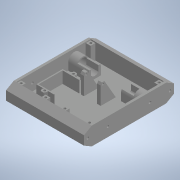
# Autodesk Inventor part: HexBody
Saved by Autodesk Inventor 2020 (Build 240168000, 168)
## iProperties
Created: 2023-12-19
Part Number: HexBody
Material: H TPU
Document SubType Name: Modeling
Designer: smz3rm
Density: 0.941117 g/cm^3
Appearance: Generic(1)
Mass: 168.679 g
Surface Area: 750.683 cm^2
Volume: 179.233 cm^3
BaseThickness: 3.000 mm
TopThickness: 1.778 mm
SideThickness: 4.000 mm
BodyWidth: 130.000 mm
BodyLength: 150.000 mm
BodyHeight: 30.000 mm
DriveMotorHeight: 15.000 mm
WheelWidth: 7.000 mm
WheelGrooveWidth: 4.000 mm
WheelGrooveDia: 16.000 mm
WheelDia: 40.000 mm
WheelPulleyDia: 2.000 mm
M3ScrewInsertBrim: 8.000 mm
M3ScrewDia: 3.100 mm
M3ScrewHeadDia: 6.100 mm
M3ScrewInsertDia: 4.000 mm
M3ScrewInsertDepth: 7.000 mm
DriveMotorOffset: 40.000 mm
DriveMotorHoleDia: 4.200 mm
M3ScrewHeadDepth: 2.200 mm
M3ScrewHeadTaper: -32.50 deg
WheeGuardlSlotWidth: 14.000 mm
WheelGuardScrewOffset: 7.000 mm
FlipperWidth: 20.000 mm
WheelSpokes: 5.000 ul
FlipperRodDia: 2.100 mm
FlipperArmThickness: 4.619 mm
FlipperArmLength: 87.010 mm
FlipperMountOffset: 70.000 mm
FlipperMountThickness: 6.000 mm
FlipperSpikeDrop: 37.509 mm
FlipperSpikeAngle: 30.00 deg
FlipperSpikeWidth: 10.000 mm
WheelGuardSpikeThickness: 8.000 mm
WheelGuardSpikeDrop: 35.200 mm
FlipperArmServoMountOffset: 30.000 mm
FlipperArmConnectorLength: 36.000 mm
Author: smz3rm
Autodesk Inventor part; units mm, degrees
ref_plane "XZ Plane" through (0, 0, 0) normal (0, 1, 0) x (-1, 0, 0)
ref_plane "XY Plane" through (0, 0, 0) normal (0, 0, 1) x (1, 0, 0)
sketch "Sketch1" plane through (0, 0, 0) normal (1, 0, 0) x (0, 1, 0)
  line L0 (-15, 75) -> (15, 75)
  line L1 (15, 75) -> (15, -75)
  line L2 (15, -75) -> (-15, -75)
  line L3 (-15, -75) -> (-15, 75)
  line L4 (-15, 75) -> (15, -75) construction
  line L5 (15, 75) -> (-15, -75) construction
  line L6 (-21, 0) -> (21, 0) projected
  line L7 (0, -105) -> (0, 105) projected
  line L8 (7.5, -75) -> (-7.5, -75)
  line L9 (-7.5, -75) -> (-15, -62.0096)
  line L10 (-15, -62.0096) -> (-7.5, -49.0192)
  line L11 (-7.5, -49.0192) -> (7.5, -49.0192)
  line L12 (7.5, -49.0192) -> (15, -62.0096)
  line L13 (15, -62.0096) -> (7.5, -75)
  line L14 (-7.5, 75) -> (-15, 62.0096)
  line L15 (15, 62.0096) -> (7.5, 75)
  point P0 (0, 0)
  point P1 (0, -62.0096)
  point P2 (7.5, 75)
  point P3 (-15, 62.0096)
  dimension "d0" = 30
  dimension "d1" = 150
  dimension "d25" = 12.9904
  constraints: 28 end point, 4 point on line, 4 symmetric about line, 2 midpoint, 2 parallel, 1 horizontal, 1 perpendicular, 13 other
  measures "d0" distance of L1.end L2.end
  measures "d1" distance of L0.end L1.end
  measures "d25" distance from line of point (0, -62.01) L2
extrude "Extrusion1" add sketch "Sketch1" along normal mid plane 130 contours L0 L7 L6 L3 L14 | L0 L15 L1 L6 L7 | L6 L7 L11 L10 L3 | L6 L1 L12 L11 L7 | L10 L11 L7 L2 L9 | L11 L12 L13 L2 L7
sketch "Sketch2" plane through (-65, 15, 62.4426) normal (0, 1, 0) x (1, 0, 0)
  line L0 (130, 124.4523) -> (130, 0.433) projected
  line L1 (0, 0.433) -> (0, 124.4523) projected
  line L2 (126, 124.4523) -> (4, 124.4523)
  line L3 (4, 124.4523) -> (4, 0.433)
  line L4 (4, 0.433) -> (126, 0.433)
  line L5 (126, 0.433) -> (126, 124.4523)
  line L6 (126, 124.4523) -> (4, 0.433) construction
  line L7 (4, 124.4523) -> (126, 0.433) construction
  line L8 (0, 0.433) -> (130, 0.433) projected
  line L9 (0, 124.4523) -> (130, 124.4523) projected
  point P0 (65, 62.4426)
  dimension "d4" = 4
  constraints: 12 end point, 2 midpoint, 2 parallel, 1 horizontal, 1 perpendicular, 1 point on line
  measures "d4" distance between parallel lines of L1 L3
extrude "Extrusion2" cut sketch "Sketch2" against normal blind 27 contours L5 L4 L3 L2
sketch "Sketch3" plane through (-65, -12, 62.4426) normal (0, 1, 0) x (1, 0, 0)
  line L0 (4, 0.433) -> (4, 124.4523) projected
  line L1 (126, 0.433) -> (4, 0.433) projected
  line L2 (126, 124.4523) -> (126, 0.433) projected
  line L3 (4, 124.4523) -> (126, 124.4523) projected
  line L4 (4, 0.433) -> (4, 124.4523) projected
  line L5 (126, 124.4523) -> (126, 0.433) projected
  line L6 (130, 124.4523) -> (130, 0.433) projected
  line L7 (0, 0.433) -> (0, 124.4523) projected
  line L8 (4, 124.4523) -> (12, 124.4523)
  line L9 (12, 124.4523) -> (12, 116.4523)
  line L10 (12, 116.4523) -> (4, 116.4523)
  line L11 (4, 116.4523) -> (4, 124.4523)
  line L12 (-26, 62.4426) -> (156, 62.4426) projected
  line L13 (65, 167.4426) -> (65, -42.5574) projected
  line L14 (118, 124.4523) -> (118, 116.4523)
  line L15 (118, 116.4523) -> (126, 116.4523)
  line L16 (12, 0.433) -> (12, 8.433)
  line L17 (12, 8.433) -> (4, 8.433)
  line L18 (118, 0.433) -> (118, 8.433)
  line L19 (118, 8.433) -> (126, 8.433)
  line L20 (0, 124.4523) -> (4, 124.4523) projected
  line L21 (0, 0.433) -> (4, 0.433) projected
  line L22 (126, 0.433) -> (130, 0.433) projected
  line L23 (126, 124.4523) -> (130, 124.4523) projected
  point P0 (65, 62.4426)
  point P1 (12, 0.433)
  point P2 (12, 124.4523)
  point P3 (118, 124.4523)
  point P4 (126, 8.433)
  point P5 (118, 0.433)
  dimension "d8" = 8
  constraints: 20 end point, 9 symmetric about line, 2 parallel, 2 perpendicular, 1 horizontal
  measures "d8" distance of L9.end L10.end
extrude "Extrusion3" add sketch "Sketch3" along normal blind 25.222 contours L0 L17 L16 L1 | L0 L3 L9 L10 | L18 L19 L2 L1 | L15 L14 L3 L2
sketch "Sketch4" plane through (-61, 15, 62.0096) normal (1, 0, 0) x (0, 0, -1)
  circle A0 centre (97.0096, -15) radius 8.25
  line L0 (124.0192, -30) -> (0, -30) projected
  line L1 (137.0096, -7.5) -> (137.0096, -22.5) projected
  circle A1 centre (97.0096, -15) radius 10.25
  line L2 (86.7596, -15) -> (86.7596, -27)
  line L3 (8, -27) -> (116.0192, -27) projected
  line L4 (107.2596, -15) -> (107.2596, -27)
  point P0 (62.0096, -15)
  dimension "d12" = 16.5
  dimension "d13" = 15
  dimension "d14" = 40
  dimension "d15" = 2
  constraints: 4 end point, 2 centre point, 2 point on circle, 2 point on line, 2 tangent, 2 vertical, 1 coincident
  measures "d12" diameter of A0
  measures "d13" distance from line of L0 A0.centre
  measures "d14" distance from line of L1 A0.centre
  measures "d15" radial gap between concentric circles of A0 A1
extrude "Extrusion4" add sketch "Sketch4" along normal blind 14
sketch "Sketch5" plane through (-47, 15, 62.0096) normal (1, 0, 0) x (0, 0, -1)
  circle A0 centre (97.0096, -15) radius 8.25 projected
  circle A1 centre (97.0096, -15) radius 7.75
  line L0 (107.2596, -27) -> (107.2596, -15) projected
  arc A2 (107.2596, -15) -> (86.7596, -15) centre (97.0096, -15) ccw projected
  line L1 (86.7596, -15) -> (86.7596, -27) projected
  line L2 (107.2596, -27) -> (86.7596, -27) projected
  circle A3 centre (97.0096, -15) radius 8.25 projected
  line L3 (90.9096, -10.2196) -> (87.9426, -10.2196)
  arc A4 (107.2596, -15) -> (86.7596, -15) centre (97.0096, -15) ccw projected
  line L4 (90.9096, -10.2196) -> (90.9096, -27)
  line L5 (107.2596, -27) -> (86.7596, -27) projected
  line L6 (103.1096, -10.2196) -> (106.0766, -10.2196)
  line L7 (103.1096, -10.2196) -> (103.1096, -27)
  point P0 (62.0096, -15)
  point P1 (90.9096, -19.7804)
  point P2 (103.1096, -19.7804)
  dimension "d18" = 15.5
  dimension "d19" = 12.2
  constraints: 8 end point, 4 point on circle, 2 horizontal, 2 perpendicular, 2 point on line, 1 centre point, 1 coincident, 1 parallel
  measures "d18" diameter of A1
  measures "d19" distance between parallel lines of L7 L4
extrude "Extrusion5" add sketch "Sketch5" along normal blind 20 contours A0 L7 A1 L6 | A0 L6 A2 L0 L2 L7 | L7 L2 L4 A0 | A0 L4 A1 L7 | L3 A1 L4 A0 | A0 L4 L2 L1 A2 L3 | A1 L7 | L4 A1
sketch "Sketch6" plane through (-61, 0, -35) normal (1, 0, 0) x (0, 0, -1)
  circle A0 centre (0, 0) radius 2.1
  point P0 (-35, 0)
  dimension "d22" = 4.2
  constraints: 1 centre point
  measures "d22" diameter of A0
extrude "Extrusion6" cut sketch "Sketch6" against normal through all
mirror "Mirror1" about plane through (0, 0, 0) normal (1, 0, 0) of "Extrusion4", "Extrusion5", "Extrusion6"
sketch "Sketch7" plane through (-65, 0, 0) normal (-1, 0, 0) x (0, 0, 1)
  line L0 (-105, 0) -> (105, 0) projected
  circle A0 centre (35, 0) radius 2
  line L1 (75, -7.5) -> (75, 7.5) projected
  point P0 (0, 0)
  dimension "d26" = 4
  dimension "d27" = 40
  constraints: 1 centre point, 1 point on line
  measures "d26" diameter of A0
  measures "d27" distance from line of L1 A0.centre
extrude "Extrusion7" cut sketch "Sketch7" against normal up to surface (4 mm away)
mirror "Mirror2" about plane through (0, 0, 0) normal (1, 0, 0) of "Extrusion7"
sketch "Sketch9" plane through (-65, 0, 0) normal (-1, 0, 0) x (0, 0, 1)
  line L0 (-62.0096, 15) -> (-62.0096, 13.222) projected
  line L1 (-62.0096, -15) -> (-62.0096, 15)
  line L2 (-75, -7.5) -> (-75, 7.5) projected
  line L3 (-75, 0) -> (-62.0096, 0)
  line L4 (-62.0096, -12) -> (-62.0096, 13.222) projected
  circle A0 centre (-68.5048, 0) radius 2
  line L5 (0, -21) -> (0, 21) projected
  circle A1 centre (68.5048, 0) radius 2
  point P0 (0, 0)
  dimension "d30" = 4
  constraints: 4 end point, 2 centre point, 2 midpoint, 1 perpendicular, 1 point on line, 1 symmetric about line, 1 vertical, 1 other
  measures "d30" diameter of A0
extrude "Extrusion8" cut sketch "Sketch9" against normal blind 7
mirror "Mirror3" about plane through (0, 0, 0) normal (1, 0, 0) of "Extrusion8"
ref_plane "Work Plane1" through (11, 0, 0) normal (1, 0, 0) x (0, 1, 0)
sketch "Sketch10" plane through (11, 0, 0) normal (1, 0, 0) x (0, 1, 0)
  line L0 (-12, 54.0096) -> (-12, -24.75) projected
  line L1 (-12, -0.9008) -> (20.8594, -0.9008)
  line L2 (20.8594, -0.9008) -> (20.8594, -7.0496)
  line L3 (20.8594, -7.0496) -> (-12, -26.021)
  circle A0 centre (17.3094, -5) radius 1.55
  line L4 (-7.5, -75) -> (7.5, -75) projected
  line L5 (15, -62.0096) -> (15, 62.0096) projected
  line L6 (-12, -24.75) -> (-12, -45.25) projected
  line L7 (-12, -24.75) -> (-12, 54.0096) projected
  line L8 (20.8594, -7.0496) -> (17.3094, -9.0992)
  line L9 (17.3094, -9.0992) -> (13.7594, -7.0496)
  line L10 (13.7594, -7.0496) -> (13.7594, -2.9504)
  line L11 (13.7594, -2.9504) -> (17.3094, -0.9008)
  line L12 (17.3094, -0.9008) -> (20.8594, -2.9504)
  line L13 (20.8594, -2.9504) -> (20.8594, -7.0496)
  point P0 (0, 0)
  point P1 (18.8594, -5)
  point P2 (15, -10.4325)
  point P3 (15, -0.9008)
  dimension "d34" = 3.1
  dimension "d38" = 70
  dimension "d40" = 1.55
  dimension "d41" = 2.3094
  dimension "d44" = 60
  dimension "d45" = 2
  constraints: 18 end point, 4 point on line, 1 coincident, 1 collinear, 1 horizontal, 1 horizontal alignment, 1 perpendicular, 15 other
  measures "d38" distance from line of L4 point (17.309, -5)
  measures "d40" distance of point (17.309, -5) point (18.859, -5)
  measures "d41" distance from line of L5 point (17.309, -5)
  measures "d44" angle of L0 L3
  measures "d45" distance from line of L13 point (18.859, -5)
extrude "Extrusion9" add sketch "Sketch10" along normal blind 6 contours L1 L5 L11 L10 L9 L3 L6 L0 | L1 L11 L5 | L12 L2 L3 L9 L5 L11 | L5 L9 L10 L11 | L5 L9 L3
mirror "Mirror4" about plane through (0, 0, 0) normal (1, 0, 0) of "Extrusion9"
sketch "Sketch12" plane through (-65, -12, 62.4426) normal (0, 1, 0) x (1, 0, 0)
  line L0 (48, 88.4636) -> (54, 88.4636) projected
  line L1 (54, 88.4636) -> (54, 63.3434) projected
  line L2 (54, 63.3434) -> (48, 63.3434) projected
  line L3 (48, 63.3434) -> (48, 88.4636) projected
  line L4 (76, 88.4636) -> (82, 88.4636) projected
  line L5 (82, 88.4636) -> (82, 63.3434) projected
  line L6 (82, 63.3434) -> (76, 63.3434) projected
  line L7 (76, 63.3434) -> (76, 88.4636) projected
  line L8 (126, 87.1926) -> (92, 87.1926) projected
  line L9 (92, 87.1926) -> (92, 107.6926) projected
  line L10 (92, 107.6926) -> (126, 107.6926) projected
  line L11 (126, 116.4523) -> (126, 107.6926) projected
  line L12 (126, 116.4523) -> (118, 116.4523) projected
  line L13 (118, 116.4523) -> (118, 124.4523) projected
  line L14 (12, 124.4523) -> (118, 124.4523) projected
  line L15 (12, 124.4523) -> (12, 116.4523) projected
  line L16 (12, 116.4523) -> (4, 116.4523) projected
  line L17 (4, 107.6926) -> (4, 116.4523) projected
  line L18 (4, 107.6926) -> (38, 107.6926) projected
  line L19 (38, 107.6926) -> (38, 87.1926) projected
  line L20 (38, 87.1926) -> (4, 87.1926) projected
  line L21 (4, 8.433) -> (4, 87.1926) projected
  line L22 (4, 8.433) -> (12, 8.433) projected
  line L23 (12, 8.433) -> (12, 0.433) projected
  line L24 (118, 0.433) -> (12, 0.433) projected
  line L25 (118, 0.433) -> (118, 8.433) projected
  line L26 (118, 8.433) -> (126, 8.433) projected
  line L27 (126, 87.1926) -> (126, 8.433) projected
  line L28 (54, 63.3434) -> (48, 63.3434) projected
  line L29 (54, 63.3434) -> (48, 63.3434) projected
  line L30 (82, 63.3434) -> (76, 63.3434) projected
  line L31 (76, 63.3434) -> (82, 63.3434) projected
  line L32 (118, 0.433) -> (12, 0.433) projected
  line L33 (53, 0.433) -> (45, 0.433)
  line L34 (45, 0.433) -> (45, 8.433)
  line L35 (45, 8.433) -> (53, 8.433)
  line L36 (53, 8.433) -> (53, 0.433)
  line L37 (65, 167.4426) -> (65, -42.5574) projected
  line L38 (85, 0.433) -> (85, 8.433)
  line L39 (85, 8.433) -> (77, 8.433)
  line L40 (77, 8.433) -> (77, 0.433)
  point P0 (65, 62.4426)
  dimension "d46" = 8
  dimension "d55" = 12
  constraints: 14 end point, 4 symmetric about line, 2 parallel, 2 perpendicular, 1 horizontal, 1 point on line
  measures "d46" distance of L34.end L35.end
  measures "d55" distance between parallel lines of L37 L36
extrude "Extrusion10" add sketch "Sketch12" along normal blind 25.222 contours L24 L40 L39 L38 | L24 L34 L35 L36
sketch "Sketch13" plane through (-65, 13.222, 62.4426) normal (0, 1, 0) x (1, 0, 0)
  line L0 (4, 116.4523) -> (4, 124.4523) projected
  line L1 (4, 116.4523) -> (12, 116.4523) projected
  line L2 (12, 116.4523) -> (12, 124.4523) projected
  line L3 (4, 124.4523) -> (12, 124.4523) projected
  line L4 (118, 124.4523) -> (126, 124.4523) projected
  line L5 (118, 124.4523) -> (118, 116.4523) projected
  line L6 (118, 116.4523) -> (126, 116.4523) projected
  line L7 (126, 124.4523) -> (126, 116.4523) projected
  line L8 (126, 8.433) -> (126, 0.433) projected
  line L9 (126, 8.433) -> (118, 8.433) projected
  line L10 (118, 8.433) -> (118, 0.433) projected
  line L11 (126, 0.433) -> (118, 0.433) projected
  line L12 (85, 0.433) -> (77, 0.433) projected
  line L13 (85, 0.433) -> (85, 8.433) projected
  line L14 (85, 8.433) -> (77, 8.433) projected
  line L15 (77, 8.433) -> (77, 0.433) projected
  line L16 (53, 0.433) -> (53, 8.433) projected
  line L17 (53, 8.433) -> (45, 8.433) projected
  line L18 (45, 8.433) -> (45, 0.433) projected
  line L19 (53, 0.433) -> (45, 0.433) projected
  line L20 (12, 0.433) -> (4, 0.433) projected
  line L21 (12, 0.433) -> (12, 8.433) projected
  line L22 (12, 8.433) -> (4, 8.433) projected
  line L23 (4, 0.433) -> (4, 8.433) projected
  line L24 (4, 124.4523) -> (126, 124.4523) projected
  line L25 (4, 116.4523) -> (12, 116.4523) projected
  line L26 (4, 0.433) -> (4, 124.4523) projected
  line L27 (12, 124.4523) -> (12, 116.4523) projected
  line L28 (8, 124.4523) -> (8, 116.4523)
  line L29 (4, 120.4523) -> (12, 120.4523)
  line L30 (65, 167.4426) -> (65, -42.5574) projected
  line L31 (156, 62.4426) -> (-26, 62.4426) projected
  circle A0 centre (8, 120.4523) radius 2
  circle A1 centre (122, 120.4523) radius 2
  circle A2 centre (8, 4.433) radius 2
  circle A3 centre (122, 4.433) radius 2
  line L32 (49, 8.433) -> (49, 0.433)
  line L33 (45, 0.433) -> (45, 8.433) projected
  line L34 (45, 4.433) -> (53, 4.433)
  line L35 (53, 8.433) -> (53, 0.433) projected
  circle A4 centre (49, 4.433) radius 2
  circle A5 centre (81, 4.433) radius 2
  point P0 (65, 62.4426)
  dimension "d51" = 4
  dimension "d52" = 4
  constraints: 8 end point, 8 midpoint, 6 centre point, 4 symmetric about line, 2 point on line, 1 parallel, 1 perpendicular, 4 other
  measures "d51" diameter of A0
  measures "d52" diameter of A4
extrude "Extrusion11" cut sketch "Sketch13" against normal blind 7 contours A0 L28 L29 | L29 L28 A0 | L28 L29 A0 | L28 A0 L29 | A4 L32 L34 | L34 L32 A4 | A4 L34 L32 | L34 A4 L32 | A1 | A2 | A3 | A5
sketch "Sketch14" plane through (-65, -12, 62.4426) normal (0, 1, 0) x (1, 0, 0)
  line L0 (18.5, 63.3434) -> (59, 63.3434)
  line L1 (59, 63.3434) -> (59, 23.3434)
  line L2 (59, 23.3434) -> (18.5, 23.3434)
  line L3 (18.5, 23.3434) -> (18.5, 63.3434)
  line L4 (61, 65.3434) -> (16.5, 65.3434)
  line L5 (16.5, 65.3434) -> (16.5, 21.3434)
  line L6 (16.5, 21.3434) -> (61, 21.3434)
  line L7 (61, 21.3434) -> (61, 65.3434)
  line L8 (48, 63.3434) -> (48, 21.3434)
  line L9 (46, 65.3434) -> (46, 21.3434)
  line L10 (36.8688, 67.3434) -> (34.5594, 63.3434)
  line L11 (34.5594, 63.3434) -> (29.9406, 63.3434)
  line L12 (29.9406, 63.3434) -> (27.6312, 67.3434)
  line L13 (27.6312, 67.3434) -> (29.9406, 71.3434)
  line L14 (29.9406, 71.3434) -> (34.5594, 71.3434)
  line L15 (34.5594, 71.3434) -> (36.8688, 67.3434)
  line L16 (18.5, 63.3434) -> (46, 63.3434)
  line L17 (32.25, 63.3434) -> (32.25, 67.3434)
  line L18 (16.5, 43.3434) -> (61, 43.3434)
  line L19 (36.8688, 19.3434) -> (34.5594, 23.3434)
  line L20 (34.5594, 23.3434) -> (29.9406, 23.3434)
  line L21 (29.9406, 23.3434) -> (27.6312, 19.3434)
  line L22 (27.6312, 19.3434) -> (29.9406, 15.3434)
  line L23 (29.9406, 15.3434) -> (34.5594, 15.3434)
  line L24 (34.5594, 15.3434) -> (36.8688, 19.3434)
  point P0 (65, 62.4426)
  point P1 (32.25, 19.3434)
  point P2 (46, 23.3434)
  point P3 (28.7859, 65.3434)
  point P4 (35.7141, 65.3434)
  point P5 (35.7141, 21.3434)
  point P6 (28.7859, 21.3434)
  dimension "d56" = 29.5
  dimension "d57" = 40
  dimension "d58" = 40.5
  dimension "d59" = 2
  dimension "d60" = 2
  dimension "d62" = 8
  constraints: 50 end point, 7 symmetric about line, 6 point on line, 4 parallel, 4 perpendicular, 3 midpoint, 1 collinear, 1 horizontal, 1 vertical, 16 other
  measures "d56" distance of L8.start L0.start
  measures "d57" distance of L2.end L0.start
  measures "d58" distance of L1.end L2.end
  measures "d59" distance between parallel lines of L0 L4
  measures "d60" distance between parallel lines of L8 L9
  measures "d62" distance between parallel lines of L11 L14
extrude "Extrusion12" add sketch "Sketch14" along normal blind 19.5 contours L3 L18 L5 L4 L12 L0 | L12 L4 L17 L0 | L3 L2 L21 L6 L5 L18 | L17 L4 L10 L0 | L12 L13 L14 L15 L10 L4 | L10 L4 L9 L0 | L2 L19 L6 L21 | L9 L6 L19 L2 | L6 L19 L24 L23 L22 L21
sketch "Sketch15" plane through (-65, 7.5, 62.4426) normal (0, 1, 0) x (1, 0, 0)
  line L0 (16.5, 21.3434) -> (28.7859, 21.3434) projected
  line L1 (46, 65.3434) -> (35.7141, 65.3434) projected
  line L2 (28.7859, 65.3434) -> (16.5, 65.3434) projected
  line L3 (16.5, 65.3434) -> (16.5, 21.3434) projected
  circle A0 centre (32.25, 67.3434) radius 2
  circle A1 centre (32.25, 19.3434) radius 2
  line L4 (29.9406, 71.3434) -> (27.6312, 67.3434) projected
  line L5 (46, 23.3434) -> (18.5, 23.3434) projected
  line L6 (18.5, 23.3434) -> (18.5, 63.3434) projected
  line L7 (18.5, 63.3434) -> (46, 63.3434) projected
  line L8 (46, 63.3434) -> (46, 65.3434) projected
  line L9 (35.7141, 65.3434) -> (36.8688, 67.3434) projected
  line L10 (36.8688, 67.3434) -> (34.5594, 71.3434) projected
  line L11 (34.5594, 71.3434) -> (29.9406, 71.3434) projected
  line L12 (29.9406, 71.3434) -> (27.6312, 67.3434) projected
  line L13 (27.6312, 67.3434) -> (28.7859, 65.3434) projected
  line L14 (28.7859, 21.3434) -> (27.6312, 19.3434) projected
  line L15 (27.6312, 19.3434) -> (29.9406, 15.3434) projected
  line L16 (29.9406, 15.3434) -> (34.5594, 15.3434) projected
  line L17 (34.5594, 15.3434) -> (36.8688, 19.3434) projected
  line L18 (36.8688, 19.3434) -> (35.7141, 21.3434) projected
  line L19 (35.7141, 21.3434) -> (46, 21.3434) projected
  line L20 (46, 21.3434) -> (46, 23.3434) projected
  line L21 (36.8688, 67.3434) -> (27.6312, 67.3434)
  line L22 (27.6312, 19.3434) -> (28.7859, 21.3434) projected
  line L23 (36.8688, 19.3434) -> (34.5594, 15.3434) projected
  line L24 (27.6312, 19.3434) -> (36.8688, 19.3434)
  point P0 (65, 62.4426)
  dimension "d65" = 4
  dimension "d66" = 4
  constraints: 4 end point, 2 centre point, 2 midpoint, 1 horizontal
  measures "d65" diameter of A0
  measures "d66" diameter of A1
extrude "Extrusion13" cut sketch "Sketch15" against normal blind 7 contours L24 A1 | A1 L24 | L21 A0 | A0 L21
sketch "Sketch16" plane through (-17, -12, -0.9008) normal (-1, 0, 0) x (0, 0, 1)
  line L0 (0, 29.3094) -> (0, 0) projected
  line L1 (0, 0) -> (-25.1202, 0) projected
  line L2 (0, 21) -> (-7.5, 21)
  line L3 (-7.5, 21) -> (-7.5, 0)
  line L4 (-7.5, 0) -> (0, 0)
  line L5 (0, 0) -> (0, 21)
  point P0 (0.9008, 12)
  dimension "d69" = 21
  dimension "d70" = 7.5
  constraints: 8 end point, 2 parallel, 2 point on line, 1 horizontal, 1 perpendicular
  measures "d69" distance of L4.end L2.start
  measures "d70" distance of L2.start L2.end
extrude "Extrusion14" cut sketch "Sketch16" against normal blind 1
equation "\"d0\" = BodyHeight"
equation "\"d1\" = BodyLength"
equation "\"d2\" = BodyWidth"
equation "\"d4\" = SideThickness"
equation "\"d5\" = BodyHeight - BaseThickness"
equation "\"d8\" = M3ScrewInsertBrim"
equation "\"d10\" = -BaseThickness + BodyHeight - TopThickness"
equation "\"d13\" = DriveMotorHeight"
equation "\"d14\" = DriveMotorOffset"
equation "\"d22\" = DriveMotorHoleDia"
equation "\"d26\" = M3ScrewInsertDia"
equation "\"d27\" = DriveMotorOffset"
equation "\"d30\" = M3ScrewInsertDia"
equation "\"d31\" = M3ScrewInsertDepth"
equation "\"d34\" = M3ScrewDia"
equation "\"d38\" = FlipperMountOffset"
equation "\"d40\" = 0.5 * d34"
equation "\"d41\" = 0.5 * FlipperArmThickness"
equation "\"d42\" = FlipperMountThickness"
equation "\"d46\" = M3ScrewInsertBrim"
equation "\"d48\" = -BaseThickness + BodyHeight - TopThickness"
equation "\"d51\" = M3ScrewInsertDia"
equation "\"d52\" = M3ScrewInsertDia"
equation "\"d53\" = M3ScrewInsertDepth"
equation "\"BaseThickness\" = 3"
equation "\"TopThickness\" = 1.778"
equation "\"SideThickness\" = 4"
equation "\"BodyWidth\" = 130"
equation "\"BodyLength\" = 150"
equation "\"BodyHeight\" = 30"
equation "\"DriveMotorHeight\" = 0.5 * BodyHeight"
equation "\"WheelWidth\" = 7"
equation "\"WheelGrooveWidth\" = 4"
equation "\"WheelGrooveDia\" = 0.4 * WheelDia"
equation "\"WheelPulleyDia\" = 2"
equation "\"M3ScrewInsertBrim\" = 8"
equation "\"M3ScrewDia\" = 3.1"
equation "\"M3ScrewHeadDia\" = 6.1"
equation "\"M3ScrewInsertDia\" = 4"
equation "\"M3ScrewInsertDepth\" = 7"
equation "\"DriveMotorOffset\" = 40"
equation "\"DriveMotorHoleDia\" = 4.2"
equation "\"M3ScrewHeadDepth\" = 2.2"
equation "\"M3ScrewHeadTaper\" = -32.5deg"
equation "\"WheelGuardScrewOffset\" = 7"
equation "\"FlipperArmLength\" = 2.5 * M3ScrewInsertBrim - FlipperMountOffset + BodyLength - 0.433013 * BodyHeight"
equation "\"FlipperWidth\" = 20"
equation "\"WheelSpokes\" = 5"
equation "\"FlipperRodDia\" = 2.1"
equation "\"FlipperMountOffset\" = 70"
equation "\"FlipperMountThickness\" = 6"
equation "\"FlipperSpikeWidth\" = 10"
equation "\"FlipperSpikeAngle\" = 30deg"
equation "\"WheelGuardSpikeThickness\" = 8"
equation "\"FlipperArmServoMountOffset\" = 30"
equation "\"FlipperArmConnectorLength\" = 36"
equation "\"WheelDia\" = 40"
equation "\"FlipperArmThickness\" = 4.618802"
body "Solid1"
